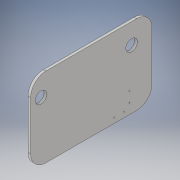
# Autodesk Inventor part: BottomRampPlate
Saved by Autodesk Inventor 2019 (Build 230136000, 136)
## iProperties
Created: 2020-01-13
Part Number: BottomRampPlate
Material: Generic
Document SubType Name: Modeling
Designer: james
Density: 1 g/cm^3
Appearance: Default
Author: james
Autodesk Inventor part; units mm, degrees
ref_plane "YZ Plane" through (0, 0, 0) normal (1, 0, 0) x (0, 1, 0)
ref_plane "XZ Plane" through (0, 0, 0) normal (0, 1, 0) x (-1, 0, 0)
ref_plane "XY Plane" through (0, 0, 0) normal (0, 0, 1) x (1, 0, 0)
sketch "Sketch1" plane through (0, 0, 0) normal (1, 0, 0) x (0, 1, 0)
  line L0 (-17.3403, 309.9338) -> (-51.2615, 309.9338)
  line L1 (-51.2615, -502.8662) -> (-17.3403, -502.8662)
  line L2 (71.5597, 7.6738) -> (193.4797, 7.6738)
  line L3 (231.5797, 45.7738) -> (231.5797, 271.8338)
  line L4 (193.4797, 309.9338) -> (71.5597, 309.9338)
  line L5 (33.4597, 271.8338) -> (33.4597, 45.7738)
  line L6 (33.4597, 50.9549) -> (33.4597, 76.3549)
  line L7 (33.4597, 119.3221) -> (33.4597, 50.9549)
  arc A0 (71.5597, 309.9338) -> (33.4597, 271.8338) centre (71.5597, 271.8338) ccw
  arc A1 (231.5797, 271.8338) -> (193.4797, 309.9338) centre (193.4797, 271.8338) ccw
  arc A2 (193.4797, 7.6738) -> (231.5797, 45.7738) centre (193.4797, 45.7738) ccw
  arc A3 (33.4597, 45.7738) -> (71.5597, 7.6738) centre (71.5597, 45.7738) ccw
  circle A4 centre (180.7797, 284.5338) radius 14.2875
  circle A5 centre (46.1597, 76.3549) radius 1.27
  circle A6 centre (46.1597, 101.7549) radius 1.27
  circle A7 centre (58.8597, 63.6549) radius 1.27
  circle A8 centre (84.2597, 63.6549) radius 1.27
  circle A9 centre (180.7797, 58.4738) radius 14.2875
  point P0 (0, 0)
  dimension "d2" = 812.8
  dimension "d17" = 302.26
  dimension "d28" = 38.1
  dimension "d29" = 28.575
  dimension "d30" = 2.54
  dimension "d32" = 12.7
  dimension "d33" = 2.54
  dimension "d34" = 12.7
  dimension "d35" = 25.4
  dimension "d36" = 0
  dimension "d37" = 2.54
  dimension "d38" = 2.54
  dimension "d40" = 25.4
  dimension "d42" = 28.575
  constraints: 16 end point, 10 centre point, 8 point on circle, 8 tangent, 3 equal radius, 3 parallel, 2 horizontal, 2 point on line, 1 perpendicular
  measures "d2" distance of L1.end L0.start
  measures "d17" distance between parallel lines of L4 L2
  measures "d28" radius of A0
  measures "d29" diameter of A4
  measures "d30" diameter of A5
  measures "d32" distance from line of L7 A5.centre
  measures "d33" diameter of A6
  measures "d34" distance from line of L7 A6.centre
  measures "d35" distance of A5.centre A6.centre
  measures "d36" vertical distance of A7.centre A8.centre
  measures "d37" diameter of A8
  measures "d38" diameter of A7
  measures "d40" distance of A8.centre A7.centre
  measures "d42" diameter of A9
extrude "Extrusion1" add sketch "Sketch1" along normal blind 6.35
body "Solid1"
